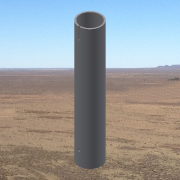
# Autodesk Inventor part: mast_paper
Saved by Autodesk Inventor 2014 SP1 (Build 180222100, 222)
## iProperties
Created: 2015-08-14
Part Number: mast_paper
Material: Generic
Document SubType Name: Modeling
Designer: Dave
Density: 1 g/cm^3
Appearance: Default
Author: Dave
Autodesk Inventor part; units mm, degrees
ref_plane "YZ Plane" through (0, 0, 0) normal (1, 0, 0) x (0, 1, 0)
ref_plane "XZ Plane" through (0, 0, 0) normal (0, 1, 0) x (-1, 0, 0)
sketch "Sketch1" plane through (0, 0, 0) normal (0, 1, 0) x (-1, 0, 0)
  circle A0 centre (0, 0) radius 44.45
  circle A1 centre (0, 0) radius 38.9636
  dimension "d0" = 88.9
  dimension "d1" = 5.4864
  constraints: 2 centre point, 1 coincident
  measures "d0" diameter of A0
  measures "d1" radial gap between concentric circles of A1 A0
extrude "Extrusion1" add sketch "Sketch1" along normal blind 481.33
ref_plane "Work Plane1" through (0, 0, 44.45) normal (0, 0, 1) x (1, 0, 0)
sketch "Sketch2" plane through (0, 0, 44.45) normal (0, 0, 1) x (1, 0, 0)
  arc A0 (-2.54, 436.88) -> (2.54, 436.88) centre (0, 436.88) ccw
  line L0 (44.45, 481.33) -> (-44.45, 481.33) projected
  line L1 (-2.54, 436.88) -> (-2.54, 481.33)
  line L2 (2.54, 436.88) -> (2.54, 481.33)
  point P0 (0, 0)
  dimension "d5" = 44.45
  dimension "d6" = 5.08
  constraints: 4 end point, 2 perpendicular, 2 point on circle, 2 point on line, 2 tangent, 1 centre point
  measures "d5" distance from line of A0.centre L0
  measures "d6" diameter of A0
extrude "Extrusion2" cut sketch "Sketch2" against normal blind 25.4
sketch "Sketch4" plane through (0, 0, 44.45) normal (0, 0, 1) x (1, 0, 0)
  line L0 (0, 54.102) -> (0, 60.452) construction
  line L1 (3.175, 54.102) -> (3.175, 60.452)
  line L2 (-3.175, 60.452) -> (-3.175, 54.102)
  arc A0 (-3.175, 54.102) -> (3.175, 54.102) centre (0, 54.102) ccw
  arc A1 (3.175, 60.452) -> (-3.175, 60.452) centre (0, 60.452) ccw
  point P0 (0, 0)
  point P1 (0, 57.277)
  dimension "d18" = 6.35
  dimension "d19" = 6.35
  dimension "d20" = 54.102
  constraints: 8 end point, 4 point on circle, 4 tangent, 2 centre point, 1 midpoint, 1 parallel, 1 vertical
  measures "d18" distance of L0.start L0.end
  measures "d19" diameter of A1
  measures "d20" distance of L0.start point (0, 0)
extrude "Extrusion3" cut sketch "Sketch4" against normal blind 25.4
sketch "Sketch5" plane through (0, 0, 0) normal (0, -1, 0) x (1, 0, 0)
  circle A0 centre (0, 0) radius 44.45 projected
  line L0 (-22.098, 38.5679) -> (-22.098, -38.5679)
  point P0 (-44.45, 0)
  dimension "d23" = 22.352
  constraints: 3 point on circle, 2 end point, 1 vertical
  measures "d23" distance from line of L0 point (-44.45, 0)
extrude "Extrusion4" cut sketch "Sketch5" against normal blind 6.35 contours L0 A0 picked at (-24.6172, 11.037)
body "Solid1"
